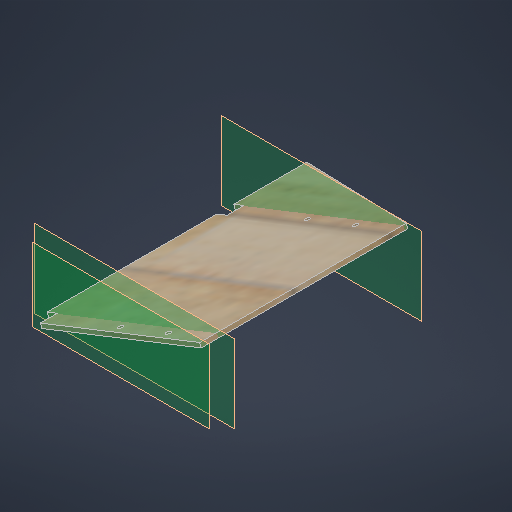
# Autodesk Inventor part: Right_Wall
Saved by Autodesk Inventor 2026.3 (Build 303398000, 398)
## iProperties
Created: 2026-09-07
Part Number: Right_Wall
Material: 木材 (カエデ材)
Document SubType Name: Modeling
Designer: takuya
Density: 0.67 g/cm^3
Appearance: ナチュラル カエデ材 - 光沢 濃い着色
Author: takuya
Autodesk Inventor part; units mm, degrees
ref_plane "YZ Plane" through (0, 0, 0) normal (1, 0, 0) x (0, 1, 0)
ref_plane "作業平面1" through (-58.5419, 13.75, 0) normal (0, 0, -1) x (-1, 0, 0)
sketch "スケッチ1" plane through (-58.5419, 13.75, 0) normal (0, 0, -1) x (-1, 0, 0)
  line L0 (-47.5988, 17.4243) -> (46.6818, -19.75) projected
  line L1 (46.6818, -19.75) -> (47.5988, -17.4243) projected
  line L2 (47.5988, -17.4243) -> (-46.6818, 19.75) projected
  line L3 (-46.6818, 19.75) -> (-47.5988, 17.4243) projected
  point P0 (-58.5419, -13.75)
ref_plane "作業平面2" through (-125.5285, -9.35, -169.7679) normal (-0.3826834, 0, 0.9238795) x (0.9238795, 0, 0.3826834)
extrude "押し出し1" add sketch "スケッチ1" along normal up to surface surface through (-125.5285, -9.35, -169.7679) normal (-0.3826834, 0, 0.9238795)
sketch "スケッチ2" plane through (-106.1408, -3.6743, 0) normal (-0.3668097, 0.930296, 0) x (0.930296, 0.3668097, 0)
  circle A0 centre (76.1355, 115.4647) radius 1.5 projected
  circle A1 centre (45.616, 115.4647) radius 1.5 projected
  line L0 (30.3562, 120.4647) -> (30.3562, 110.4647) projected
  line L1 (91.3953, 120.4647) -> (30.3562, 120.4647) projected
  line L2 (91.3953, 110.4647) -> (91.3953, 120.4647) projected
  line L3 (30.3562, 110.4647) -> (91.3953, 110.4647) projected
  circle A2 centre (76.1355, 5) radius 1.5 projected
  circle A3 centre (45.616, 5) radius 1.5 projected
  line L4 (30.3562, 10) -> (30.3562, 0) projected
  line L5 (91.3953, 10) -> (30.3562, 10) projected
  line L6 (91.3953, 0) -> (91.3953, 10) projected
  line L7 (30.3562, 0) -> (91.3953, 0) projected
  point P0 (100.0901, 0)
extrude "押し出し2" cut sketch "スケッチ2" against normal blind 10 contours A0 | A1 | A2 | A3
ref_plane "作業平面3" through (-60.4061, 12.6229, -10) normal (0, 0, -1) x (-1, 0, 0)
sketch "スケッチ3" plane through (-60.4061, 12.6229, -10) normal (0, 0, -1) x (-1, 0, 0)
  line L0 (53.8577, -19.5) -> (45.423, -16.1743)
  line L1 (53.8577, -21) -> (53.8577, -19.5)
  line L2 (-53.8577, -21) -> (53.8577, -21)
  line L3 (44.8176, -18.6229) -> (45.7346, -16.2971) projected
  line L4 (45.7346, -16.2971) -> (44.8176, -18.6229)
  line L5 (44.8176, -18.6229) -> (50.8464, -21)
  line L6 (50.8464, -21) -> (51.7634, -18.6743)
  line L7 (51.7634, -18.6743) -> (45.7346, -16.2971)
  point P0 (-60.4061, -12.6229)
  point P1 (44.506, -18.5)
  point P2 (51.7634, -18.6743)
  constraints: 14 end point, 3 equal length, 1 horizontal, 1 perpendicular, 1 point on line, 1 vertical, 6 other
ref_plane "作業平面4" through (-114.2638, -8.3771, -110.4647) normal (0, 0, 1) x (1, 0, 0)
extrude "押し出し3" add sketch "スケッチ3" along normal up to surface (100.4647 mm away) contours L6 L5 L3 L0
ref_plane "作業平面5" through (-60.4061, 12.6229, -120.4647) normal (0, 0, -1) x (-1, 0, 0)
sketch "スケッチ4" plane through (-60.4061, 12.6229, -120.4647) normal (0, 0, -1) x (-1, 0, 0)
  line L0 (50.8464, -21) -> (51.7634, -18.6743) projected
  line L1 (44.8176, -18.6229) -> (45.7346, -16.2971) projected
  line L2 (53.8577, -19.5) -> (45.423, -16.1743)
  line L3 (44.8176, -18.6229) -> (50.8464, -21) projected
  point P0 (-60.4061, -12.6229)
  constraints: 2 end point, 3 other
extrude "押し出し4" add sketch "スケッチ4" along normal up to surface surface through (-58.5419, 13.75, -142.0212) normal (-0.3826834, 0, 0.9238795)
sketch "スケッチ6" plane through (-11.8601, 33.5, 0) normal (-0.3668097, 0.930296, 0) x (0.930296, 0.3668097, 0)
  line L0 (-107.8253, 164.2345) -> (0, 122.685) projected
  line L1 (0, 0) -> (0, 122.685) projected
  line L2 (-107.8253, 120.4647) -> (-107.8253, 164.2345) projected
  line L3 (-107.8253, 163.6987) -> (0, 122.1491)
  point P0 (-1.2547, 0)
  dimension "d9" = 0.5
  constraints: 2 end point, 2 point on line, 1 parallel
  measures "d9" distance between parallel lines of L3 L0
extrude "押し出し5" cut sketch "スケッチ6" against normal blind 2.5
